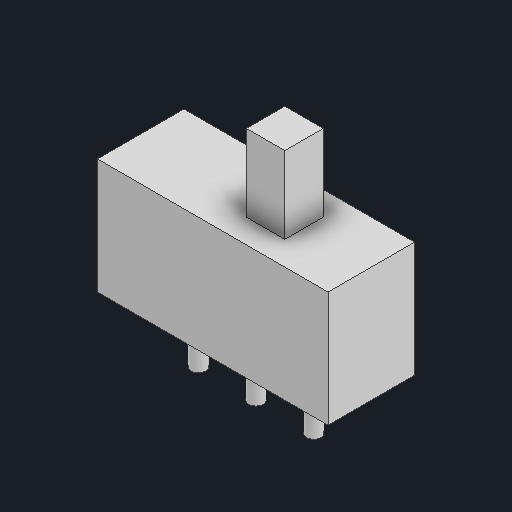
# Autodesk Inventor part: tmdnlcl
Saved by Autodesk Inventor 2027.1 (Build 311270010, 270A)
## iProperties
Created: 2026-08-07
Part Number: tmdnlcl
Material: 일반
Document SubType Name: Modeling
Designer: moieboy9999
Density: 2.90718 g/cm^3
Appearance: 기본값
Mass: 1 g
Surface Area: 3.59206 cm^2
Volume: 0.343976 cm^3
Author: moieboy9999
Autodesk Inventor part; units mm, degrees
ref_plane "YZ Plane" through (0, 0, 0) normal (1, 0, 0) x (0, 1, 0)
ref_plane "XZ Plane" through (0, 0, 0) normal (0, 1, 0) x (-1, 0, 0)
ref_plane "XY Plane" through (0, 0, 0) normal (0, 0, 1) x (1, 0, 0)
sketch "스케치4" plane through (0, 0, 0) normal (0, 1, 0) x (-1, 0, 0)
  line L0 (0, 0) -> (-12, 0)
  line L1 (-12, 0) -> (-12, -4.5)
  line L2 (-12, -4.5) -> (0, -4.5)
  line L3 (0, -4.5) -> (0, 0)
  dimension "d18" = 12
  dimension "d19" = 4.5
  constraints: 8 end point, 2 parallel, 1 horizontal, 1 perpendicular
  measures "d18" distance of L2.end L1.end
  measures "d19" distance of L1.end L0.end
extrude "돌출5" add sketch "스케치4" along normal blind 6
sketch "스케치5" plane through (0, 6, 0) normal (0, 1, 0) x (1, 0, 0)
  line L0 (12, 0) -> (12, 4.5) projected
  line L1 (12, 2.25) -> (12, 3.25)
  line L2 (12, 3.25) -> (6.5, 3.25)
  line L3 (6.5, 3.25) -> (8.5, 3.25)
  line L4 (8.5, 3.25) -> (8.5, 1.25)
  line L5 (8.5, 1.25) -> (6.5, 1.25)
  line L6 (6.5, 1.25) -> (6.5, 3.25)
  point P0 (0, 0)
  dimension "d22" = 1
  dimension "d23" = 5.5
  dimension "d24" = 2
  dimension "d25" = 2
  constraints: 12 end point, 2 parallel, 2 perpendicular, 1 horizontal, 1 midpoint, 1 point on line
  measures "d22" distance of L1.start L1.end
  measures "d23" distance of L1.end L2.end
  measures "d24" distance of L4.end L5.end
  measures "d25" distance of L3.end L4.end
extrude "돌출6" add sketch "스케치5" along normal blind 4
sketch "스케치6" plane through (0, 0, 0) normal (0, -1, 0) x (1, 0, 0)
  line L0 (0, 0) -> (12, 0) projected
  line L1 (6, 0) -> (6, -2.25)
  line L2 (6, -2.25) -> (9, -2.25)
  line L3 (9, -2.25) -> (3, -2.25)
  circle A0 centre (6, -2.25) radius 0.375
  circle A1 centre (9, -2.25) radius 0.375
  circle A2 centre (3, -2.25) radius 0.375
  dimension "d28" = 2.25
  dimension "d29" = 3
  dimension "d30" = 6
  dimension "d31" = 0.75
  dimension "d32" = 0.75
  dimension "d33" = 0.75
  constraints: 6 end point, 3 centre point, 3 coincident, 1 midpoint, 1 perpendicular, 1 point on line, 1 vertical
  measures "d28" distance of L1.start L1.end
  measures "d29" distance of L1.end L2.end
  measures "d30" distance of L2.end L3.end
  measures "d31" diameter of A0
  measures "d32" diameter of A1
  measures "d33" diameter of A2
extrude "돌출7" add sketch "스케치6" along normal blind 3
